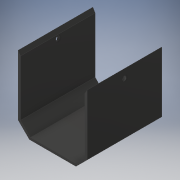
# Autodesk Inventor part: A03
Saved by Autodesk Inventor 2017 (Build 210142000, 142)
## iProperties
Created: 2019-11-14
Part Number: A03
Material: ABS Plastic
Document SubType Name: Modeling
Designer: Zach
Density: 1.06 g/cm^3
Appearance: Smooth - Black
Mass: 320.955 g
Surface Area: 704.158 cm^2
Volume: 302.787 cm^3
Author: Zach
Autodesk Inventor part; units mm, degrees
ref_plane "YZ Plane" through (0, 0, 0) normal (1, 0, 0) x (0, 1, 0)
ref_plane "XZ Plane" through (0, 0, 0) normal (0, 1, 0) x (-1, 0, 0)
ref_plane "XY Plane" through (0, 0, 0) normal (0, 0, 1) x (1, 0, 0)
sketch "Sketch1" plane through (0, 0, 0) normal (0, 0, 1) x (1, 0, 0)
  line L0 (-46.188, 0) -> (-23.094, 40)
  line L1 (-23.094, 40) -> (23.094, 40)
  line L2 (23.094, 40) -> (46.188, 0)
  line L3 (46.188, 0) -> (23.094, -40)
  line L4 (23.094, -40) -> (-23.094, -40)
  line L5 (-23.094, -40) -> (-46.188, 0)
  line L6 (-48.188, 0) -> (-46.188, 0)
  line L7 (46.188, 0) -> (48.188, 0)
  line L8 (-46.188, 0) -> (-43.188, -5.1962)
  line L9 (46.188, 0) -> (43.188, -5.1962)
  line L10 (-46.188, 0) -> (-46.188, -81)
  line L11 (-46.188, -81) -> (-31.188, -96)
  line L12 (-31.188, -96) -> (31.188, -96)
  line L13 (31.188, -96) -> (46.188, -81)
  line L14 (46.188, -81) -> (46.188, 0)
  line L15 (43.188, -5.1962) -> (43.188, -79.7574)
  line L16 (43.188, -79.7574) -> (29.9454, -93)
  line L17 (29.9454, -93) -> (-29.9454, -93)
  line L18 (-29.9454, -93) -> (-43.188, -79.7574)
  line L19 (-43.188, -79.7574) -> (-43.188, -5.1962)
  point P0 (0, 0)
  point P1 (0, 0)
  point P2 (0, -96)
  dimension "d0" = 80
  dimension "d6" = 56
  dimension "d7" = 15
  dimension "d8" = 15
  dimension "d9" = 3
  constraints: 40 end point, 3 horizontal, 2 parallel, 2 perpendicular, 2 point on line, 1 coincident, 1 horizontal alignment, 1 midpoint, 1 vertical, 1 vertical alignment, 17 other
  measures "d0" distance between parallel lines of L4 L1
  measures "d6" distance between parallel lines of L12 L4
  measures "d7" horizontal distance of L10.end L11.end
  measures "d8" horizontal distance of L11.end L10.end
  measures "d9" distance between parallel lines of L11 L18
extrude "Extrusion1" add sketch "Sketch1" along normal blind 100 contours L5 L19 L18 L17 L16 L15 L3 L14 L13 L12 L11 L10
sketch "Sketch2" plane through (-46.188, 0, 100) normal (0.866, 0.5, 0) x (0, 0, -1)
  circle A0 centre (50, -10) radius 2.5
  line L0 (100, 0) -> (0, 0) projected
  point P0 (100, -23.094)
  point P1 (50, 0)
  dimension "d10" = 5
  dimension "d11" = 10
  constraints: 1 centre point, 1 midpoint, 1 vertical alignment
  measures "d10" diameter of A0
  measures "d11" distance from line of L0 A0.centre
extrude "Extrusion2" cut sketch "Sketch2" against normal through all
sketch "Sketch3" plane through (43.188, -5.1962, 0) normal (-0.866, 0.5, 0) x (0, 0, 1)
  circle A0 centre (50, -4) radius 2.5
  line L0 (0, 6) -> (100, 6) projected
  point P0 (0, -17.094)
  point P1 (50, 6)
  dimension "d14" = 5
  dimension "d15" = 10
  constraints: 1 centre point, 1 midpoint, 1 vertical alignment
  measures "d14" diameter of A0
  measures "d15" distance from line of L0 A0.centre
extrude "Extrusion3" cut sketch "Sketch3" against normal through all
body "Solid1"
